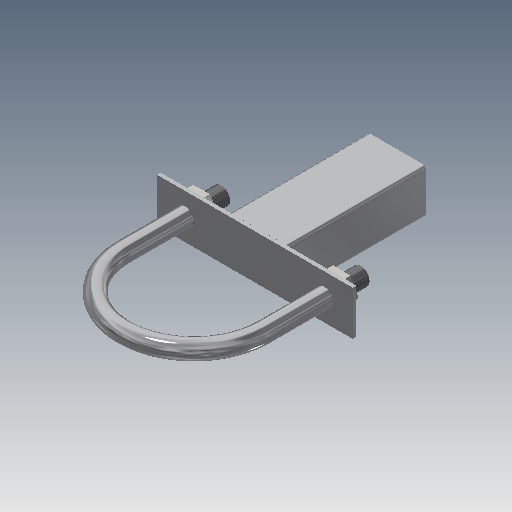
# Autodesk Inventor part: Pipe Support Valve U-Ring
Saved by Autodesk Inventor 2020 (Build 240152000, 152)
## iProperties
Created: 2007-10-29
Part Number: Pipe Support Valve U-Ring
Material: Stainless Steel
Document SubType Name: Modeling
Designer: Demir Ali
Mass: 4268.72 g
Surface Area: 1880.89 cm^2
Volume: 533.589 cm^3
Density: 8 g/cm^3
Appearance: Aluminum - Polished
Description: Pipe Support
Stock Number: NA
Author: Demir Ali
Title: Manufactured Part
Revision Number: A
Autodesk Inventor part; units mm, degrees
ref_plane "YZ Plane" through (0, 0, 0) normal (1, 0, 0) x (0, 1, 0)
sketch "Sketch1" plane through (0, 0, 0) normal (0, 1, 0) x (-1, 0, 0)
  arc A0 (-82.5, 275) -> (82.5, 275) centre (0, 275) ccw construction
  line L0 (82.5, 192.5) -> (-82.5, 192.5) construction
  line L1 (82.5, 275) -> (82.5, 142.5)
  line L2 (-82.5, 275) -> (-82.5, 142.5)
  arc A1 (82.5, 275) -> (-82.5, 275) centre (0, 275) ccw
  line L3 (82.5, 142.5) -> (-82.5, 142.5) construction
  point P0 (0, 0)
  dimension "Thread" = 50
  dimension "d13" = 275
  constraints: 8 end point, 4 point on circle, 3 perpendicular, 3 tangent, 3 vertical alignment, 2 centre point, 2 point on line, 1 horizontal, 1 other
  measures "Thread" distance between parallel lines of L3 L0
  measures "d13" distance of point (0, 0) A0.centre
ref_plane "Work Plane1" through (-82.5, 0, 142.5) normal (0, 0, -1) x (-1, 0, 0)
sketch "Sketch2" plane through (-82.5, 0, 142.5) normal (0, 0, -1) x (-1, 0, 0)
  circle A0 centre (12, 0) radius 12
  point P0 (-82.5, 0)
  point P1 (0, 0)
  dimension "d2" = 24
  constraints: 2 horizontal alignment, 2 other
sweep "Sweep1" add profiles "Sketch2" path "Sketch1"
thread "Thread1"
thread "Thread2"
chamfer "Chamfer1" distance 1 angle 45 4 edges at (82.5, 0, 142.5) (82.5, 0, 275) (-82.5, 0, 275) (-82.5, 0, 142.5)
ref_plane "Work Plane3" through (-82.5, 0, 192.5) normal (0, 0, 1) x (1, 0, 0)
sketch "Sketch3" plane through (-82.5, 0, 192.5) normal (0, 0, 1) x (1, 0, 0)
  line L0 (215, -30) -> (-50, -30)
  line L1 (-50, -30) -> (-50, 30)
  line L2 (-50, 30) -> (215, 30)
  line L3 (215, 30) -> (215, -30)
  line L4 (215, -30) -> (-50, 30) construction
  line L5 (-50, -30) -> (215, 30) construction
  circle A0 centre (-12, 0) radius 12 projected
  circle A1 centre (177, 0) radius 12 projected
  line L6 (117.5, -30) -> (47.5, -30)
  line L7 (42.5, -25) -> (42.5, 25)
  line L8 (47.5, 30) -> (117.5, 30)
  line L9 (122.5, 25) -> (122.5, -25)
  line L10 (122.5, -30) -> (42.5, 30) construction
  line L11 (42.5, -30) -> (122.5, 30) construction
  arc A2 (42.5, -25) -> (47.5, -30) centre (47.5, -25) ccw
  arc A3 (47.5, 30) -> (42.5, 25) centre (47.5, 25) ccw
  arc A4 (122.5, 25) -> (117.5, 30) centre (117.5, 25) ccw
  arc A5 (117.5, -30) -> (122.5, -25) centre (117.5, -25) ccw
  line L12 (46, 25) -> (46, -25)
  arc A6 (46, -25) -> (47.5, -26.5) centre (47.5, -25) ccw
  line L13 (47.5, -26.5) -> (117.5, -26.5)
  arc A7 (117.5, -26.5) -> (119, -25) centre (117.5, -25) ccw
  line L14 (119, -25) -> (119, 25)
  arc A8 (119, 25) -> (117.5, 26.5) centre (117.5, 25) ccw
  line L15 (117.5, 26.5) -> (47.5, 26.5)
  arc A9 (47.5, 26.5) -> (46, 25) centre (47.5, 25) ccw
  line L16 (0.1619, -19.6321) -> (-22.921, -20.3486)
  line L17 (-22.921, -20.3486) -> (-35.0829, -0.7165)
  line L18 (-35.0829, -0.7165) -> (-24.1619, 19.6321)
  line L19 (-24.1619, 19.6321) -> (-1.079, 20.3486)
  line L20 (-1.079, 20.3486) -> (11.0829, 0.7165)
  line L21 (11.0829, 0.7165) -> (0.1619, -19.6321)
  point P0 (82.5, 0)
  point P1 (-12, 0)
  dimension "d15" = 265
  dimension "d16" = 60
  dimension "d21" = 80
  dimension "d22" = 60
  dimension "d23" = 5
  dimension "d24" = 3.5
  dimension "d27" = 40
  constraints: 44 end point, 16 point on circle, 8 centre point, 8 point on line, 8 tangent, 6 parallel, 4 midpoint, 3 equal radius, 3 perpendicular, 2 horizontal, 1 coincident, 20 other
  measures "d15" distance of L1.end L2.end
  measures "d16" distance of L0.end L1.end
  measures "d21" distance of L10.end L11.end
  measures "d22" distance of L11.start L10.end
  measures "d23" radius of A2
  measures "d24" distance between parallel lines of L7 L12
  measures "d27" distance between parallel lines of L19 L16
extrude "Extrusion1" add sketch "Sketch3" against normal blind 5 separate body contours L0 A5 L9 A4 L2 L3 | L0 A2 L7 A3 L2 A4 L9 A5 | L0 L1 L2 A3 L7 A2 | A0 | A1 | A9 L15 A8 L14 A7 L13 A6 L12 | L16 L17 L18 L19 L20 L21
extrude "Extrusion2" cut sketch "Sketch3" against normal through all contours A0 | A1 bodies 2
extrude "Extrusion3" add sketch "Sketch3" against normal up to surface (187.5 mm away) from surface at -5 separate body contours L0 A2 L7 A3 L2 A4 L9 A5
extrude "Extrusion4" add sketch "Sketch3" against normal blind 18 from surface at -5 separate body contours L16 L17 L18 L19 L20 L21
mirror "Mirror1" about plane through (0, 0, 0) normal (1, 0, 0) bodies 4
equation "\"d4\" = Thread"
equation "\"d6\" = Thread"
body "Solid1"
body "Solid2"
body "Solid3"
body "Solid4"
body "Solid5"
